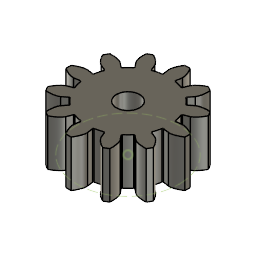
GarraGS-MakerLab_ (Autodesk Fusion 360 archive; units mm, degrees)
design "Spur Gear 12 teeth"
description: Spur Gear; Module: 1.1; Num Teeth: 12; Pressure Angle: 20.0; Backlash: 0.00 mm
part number: 2026-06-03-12-49-42-314
Autodesk Fusion 360 part; units mm, degrees
sketch "Esboço1" plane through (0, 0, 0) normal (0, 0, 1) x (1, 0, 0)
  circle A0 centre (0, 0) radius 5.3273
  circle A1 centre (0, 0) radius 1.5
extrude "Extrusão1" add sketch "Esboço1" along normal blind 6
sketch "Esboço2" plane through (0, 0, 0) normal (0, 0, 1) x (1, 0, 0)
  spline S0 degree 5 poles (6.1362, -0.9011) (6.1405, -0.9017) (6.1493, -0.9029) (6.1624, -0.9042) (6.18, -0.9051) (6.202, -0.9052) (6.2242, -0.9045) (6.2464, -0.9033) (6.2686, -0.9019) (6.2909, -0.9002) (6.3132, -0.8984) (6.3355, -0.8963) (6.3578, -0.8939) (6.3802, -0.8912) (6.4026, -0.888) (6.425, -0.8845) (6.4474, -0.8806) (6.4699, -0.8765) (6.4923, -0.8722) (6.5148, -0.8676) (6.5373, -0.8629) (6.5598, -0.8579) (6.5822, -0.8526) (6.6047, -0.8471) (6.6272, -0.8414) (6.6497, -0.8354) (6.6722, -0.8292) (6.6947, -0.8228) (6.7172, -0.8162) (6.7397, -0.8093) (6.7622, -0.8023) (6.7847, -0.795) (6.8072, -0.7876) (6.8297, -0.7799) (6.8521, -0.7721) (6.8746, -0.764) (6.8971, -0.7558) (6.9195, -0.7474) (6.9419, -0.7387) (6.9644, -0.7299) (6.9868, -0.7209) (7.0092, -0.7117) (7.0315, -0.7023) (7.0539, -0.6928) (7.0763, -0.683) (7.0986, -0.6731) (7.1209, -0.663) (7.1432, -0.6527) (7.1655, -0.6423) (7.1877, -0.6317) (7.21, -0.6209) (7.2322, -0.6099) (7.2544, -0.5988) (7.2765, -0.5874) (7.2987, -0.576) (7.3208, -0.5643) (7.3429, -0.5525) (7.365, -0.5405) (7.387, -0.5284) (7.409, -0.516) (7.431, -0.5036) (7.453, -0.4909) (7.4749, -0.4781) (7.4968, -0.4652) (7.5187, -0.452) (7.5405, -0.4388) (7.5623, -0.4253) (7.5841, -0.4117) (7.6058, -0.398) (7.6275, -0.3841) (7.6492, -0.37) (7.6665, -0.3586) (7.6795, -0.35) (7.6881, -0.3443) (7.6924, -0.3414) knots 0 0 0 0 0 0 0.01428571 0.02857143 0.04285714 0.05714286 0.07142857 0.08571429 0.1 0.11428571 0.12857143 0.14285714 0.15714286 0.17142857 0.18571429 0.2 0.21428571 0.22857143 0.24285714 0.25714286 0.27142857 0.28571429 0.3 0.31428571 0.32857143 0.34285714 0.35714286 0.37142857 0.38571429 0.4 0.41428571 0.42857143 0.44285714 0.45714286 0.47142857 0.48571429 0.5 0.51428571 0.52857143 0.54285714 0.55714286 0.57142857 0.58571429 0.6 0.61428571 0.62857143 0.64285714 0.65714286 0.67142857 0.68571429 0.7 0.71428571 0.72857143 0.74285714 0.75714286 0.77142857 0.78571429 0.8 0.81428571 0.82857143 0.84285714 0.85714286 0.87142857 0.88571429 0.9 0.91428571 0.92857143 0.94285714 0.95714286 0.97142857 0.98571429 1 1 1 1 1 1
  spline S1 degree 5 poles (6.1362, 0.9011) (6.1405, 0.9017) (6.1493, 0.9029) (6.1624, 0.9042) (6.18, 0.9051) (6.202, 0.9052) (6.2242, 0.9045) (6.2464, 0.9033) (6.2686, 0.9019) (6.2909, 0.9002) (6.3132, 0.8984) (6.3355, 0.8963) (6.3578, 0.8939) (6.3802, 0.8912) (6.4026, 0.888) (6.425, 0.8845) (6.4474, 0.8806) (6.4699, 0.8765) (6.4923, 0.8722) (6.5148, 0.8676) (6.5373, 0.8629) (6.5598, 0.8579) (6.5822, 0.8526) (6.6047, 0.8471) (6.6272, 0.8414) (6.6497, 0.8354) (6.6722, 0.8292) (6.6947, 0.8228) (6.7172, 0.8162) (6.7397, 0.8093) (6.7622, 0.8023) (6.7847, 0.795) (6.8072, 0.7876) (6.8297, 0.7799) (6.8521, 0.7721) (6.8746, 0.764) (6.8971, 0.7558) (6.9195, 0.7474) (6.9419, 0.7387) (6.9644, 0.7299) (6.9868, 0.7209) (7.0092, 0.7117) (7.0315, 0.7023) (7.0539, 0.6928) (7.0763, 0.683) (7.0986, 0.6731) (7.1209, 0.663) (7.1432, 0.6527) (7.1655, 0.6423) (7.1877, 0.6317) (7.21, 0.6209) (7.2322, 0.6099) (7.2544, 0.5988) (7.2765, 0.5874) (7.2987, 0.576) (7.3208, 0.5643) (7.3429, 0.5525) (7.365, 0.5405) (7.387, 0.5284) (7.409, 0.516) (7.431, 0.5036) (7.453, 0.4909) (7.4749, 0.4781) (7.4968, 0.4652) (7.5187, 0.452) (7.5405, 0.4388) (7.5623, 0.4253) (7.5841, 0.4117) (7.6058, 0.398) (7.6275, 0.3841) (7.6492, 0.37) (7.6665, 0.3586) (7.6795, 0.35) (7.6881, 0.3443) (7.6924, 0.3414) knots 0 0 0 0 0 0 0.01428571 0.02857143 0.04285714 0.05714286 0.07142857 0.08571429 0.1 0.11428571 0.12857143 0.14285714 0.15714286 0.17142857 0.18571429 0.2 0.21428571 0.22857143 0.24285714 0.25714286 0.27142857 0.28571429 0.3 0.31428571 0.32857143 0.34285714 0.35714286 0.37142857 0.38571429 0.4 0.41428571 0.42857143 0.44285714 0.45714286 0.47142857 0.48571429 0.5 0.51428571 0.52857143 0.54285714 0.55714286 0.57142857 0.58571429 0.6 0.61428571 0.62857143 0.64285714 0.65714286 0.67142857 0.68571429 0.7 0.71428571 0.72857143 0.74285714 0.75714286 0.77142857 0.78571429 0.8 0.81428571 0.82857143 0.84285714 0.85714286 0.87142857 0.88571429 0.9 0.91428571 0.92857143 0.94285714 0.95714286 0.97142857 0.98571429 1 1 1 1 1 1
  arc A0 (7.6924, -0.3414) -> (7.6924, 0.3414) centre (0, 0) ccw
  line L0 (5.2609, -0.7725) -> (6.1362, -0.9011)
  line L1 (5.2609, 0.7725) -> (6.1362, 0.9011)
  line L2 (5.2609, -0.7725) -> (5.2609, 0.7725)
  point P0 (6.244, -0.9034)
  point P1 (6.3533, -0.8944)
  point P2 (6.4637, -0.8776)
  point P3 (6.5747, -0.8543)
  point P4 (6.6863, -0.8252)
  point P5 (6.7982, -0.7906)
  point P6 (6.9103, -0.7508)
  point P7 (7.0226, -0.7061)
  point P8 (7.1348, -0.6566)
  point P9 (7.247, -0.6024)
  point P10 (7.3589, -0.5438)
  point P11 (7.4705, -0.4806)
  point P12 (7.5817, -0.4132)
  point P13 (6.244, 0.9034)
  point P14 (6.3533, 0.8944)
  point P15 (6.4637, 0.8776)
  point P16 (6.5747, 0.8543)
  point P17 (6.6863, 0.8252)
  point P18 (6.7982, 0.7906)
  point P19 (6.9103, 0.7508)
  point P20 (7.0226, 0.7061)
  point P21 (7.1348, 0.6566)
  point P22 (7.247, 0.6024)
  point P23 (7.3589, 0.5438)
  point P24 (7.4705, 0.4806)
  point P25 (7.5817, 0.4132)
extrude "Extrusão2" add sketch "Esboço2" along normal blind 6
fillet "Arredondamento1" radius 0.1 2 edges at (5.2708, -0.774, 3) (5.2708, 0.774, 3)
pattern_circular "Padrão circular1" count 12 over 360 about axis through (0, 0, 0) along (0, 0, 1) of "Extrusão2", "Arredondamento1"
sketch "Esboço3" plane through (0, 0, 0) normal (0, 0, 1) x (1, 0, 0)
  circle A0 centre (0, 0) radius 6.6 construction
